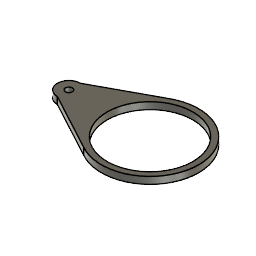
dcmountmay25 (Autodesk Fusion 360 design; units mm, degrees)
Autodesk Fusion 360 part; units mm, degrees
sketch "Sketch1" plane through (0, 0, 0) normal (0, 0, 1) x (1, 0, 0)
  circle A0 centre (0, 0) radius 1.5
  circle A1 centre (35, 0) radius 18.5
  circle A2 centre (0, 0) radius 5
  circle A3 centre (35, 0) radius 21
  line L0 (0, -5) -> (24.6535, -18.2743)
  line L1 (0, 5) -> (24.6535, 18.2743)
  dimension "d1" = 3
  dimension "d2" = 37
  dimension "d3" = 35
  dimension "d4" = 10
  dimension "d7" = 42
  dimension "d8" = 28
  dimension "d9" = 28
  constraint coincident A0.centre A2.centre
  constraint horizontal A0.centre A1.centre
  constraint concentric A0 A2
  constraint concentric A1 A3
  constraint coincident A2 L0.start
  constraint coincident A3 L0.end
  constraint coincident A2 L1.start
  constraint coincident A3 L1.end
  constraint vertical A0.centre L1.start
  constraint vertical A0.centre L0.start
  measures "d1" diameter of A0
  measures "d2" diameter of A1
  measures "d3" horizontal distance of A0.centre A1.centre
  measures "d4" diameter of A2
  measures "d7" diameter of A3
  measures "d8" distance of L1.start L1.end
  measures "d9" distance of L0.start L0.end
extrude "Extrude1" add sketch "Sketch1" along normal blind 3
